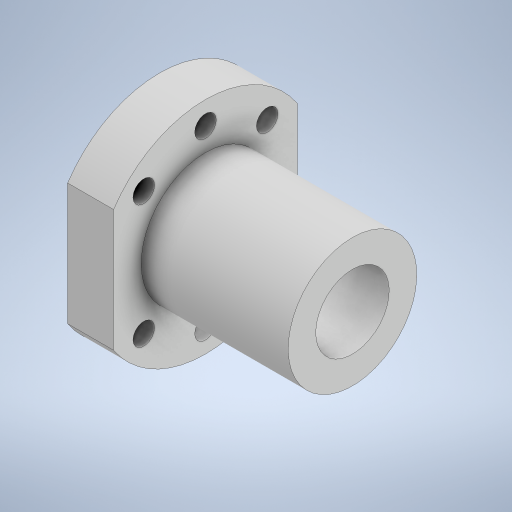
# Autodesk Inventor part: SFU1605_Nut
Saved by Autodesk Inventor 2023 (Build 270158000, 158)
## iProperties
Created: 2022-05-01
Part Number: SFU1605_Nut
Material: Generic
Document SubType Name: Modeling
Designer: plebbb
Density: 1 g/cm^3
Appearance: Default
Author: plebbb
Autodesk Inventor part; units mm, degrees
ref_plane "YZ Plane" through (0, 0, 0) normal (1, 0, 0) x (0, 1, 0)
ref_plane "XZ Plane" through (0, 0, 0) normal (0, 1, 0) x (-1, 0, 0)
ref_plane "XY Plane" through (0, 0, 0) normal (0, 0, 1) x (1, 0, 0)
sketch "Sketch1" plane through (0, 0, 0) normal (0, 0, 1) x (1, 0, 0)
  line L0 (0, 24) -> (10, 24)
  line L1 (10, 24) -> (10, 14)
  line L2 (0, 24) -> (0, 8)
  line L3 (0, 8) -> (42, 8)
  line L4 (42, 8) -> (42, 14)
  line L5 (42, 14) -> (10, 14)
  line L6 (-8.4, 0) -> (50.4, 0) projected
  point P0 (0, 0)
  point P1 (0, 16)
  dimension "d0" = 8
  dimension "d1" = 14
  dimension "d2" = 24
  dimension "d3" = 10
  dimension "d4" = 42
  constraints: 12 end point, 4 perpendicular, 2 vertical, 1 midpoint, 1 vertical alignment
  measures "d0" distance of point (0, 0) L2.end
  measures "d1" distance from line of point (0, 0) L5
  measures "d2" distance from line of point (0, 0) L0
  measures "d3" distance of L0.start L0.end
  measures "d4" distance between parallel lines of L2 L4
revolve "Revolution1" add sketch "Sketch1" angle 360 about axis through (-10, 0, 0) along (1, 0, 0)
sketch "Sketch2" plane through (0, 0, 0) normal (-1, 0, 0) x (0, 0, 1)
  circle A0 centre (0, 0) radius 19 construction
  line L0 (-20, 13.2665) -> (-20, -13.2665)
  circle A1 centre (0, 0) radius 24 projected
  line L1 (20, -13.2665) -> (20, 13.2665)
  circle A2 centre (0, 0) radius 24 projected
  circle A3 centre (-13.435, 13.435) radius 2.35
  circle A4 centre (0, 19) radius 2.35
  circle A5 centre (13.435, 13.435) radius 2.35
  circle A6 centre (-13.435, -13.435) radius 2.35
  circle A7 centre (13.435, -13.435) radius 2.35
  circle A8 centre (0, -19) radius 2.35
  line L2 (0, 0) -> (13.435, 13.435)
  line L3 (0, 0) -> (0, 19)
  dimension "d6" = 38
  dimension "d7" = 40
  dimension "d8" = 4.7
  dimension "d9" = 45
  constraints: 12 point on circle, 8 end point, 7 centre point, 5 equal radius, 3 horizontal alignment, 3 vertical alignment, 1 coincident, 1 parallel, 1 vertical
  measures "d6" diameter of A0
  measures "d7" distance between parallel lines of L1 L0
  measures "d8" diameter of A3
  measures "d9" angle of L2 L3
extrude "Extrusion1" cut sketch "Sketch2" against normal blind 10 contours L0 A1 | A1 L1 | A3 | A4 | A5 | A6 | A7 | A8
body "Solid1"
